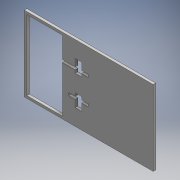
# Autodesk Inventor part: Lag2
Saved by Autodesk Inventor 2016 (Build 200138000, 138)
## iProperties
Created: 2016-12-11
Part Number: Lag2
Material: Generic
Document SubType Name: Modeling
Designer: Simon
Density: 1 g/cm^3
Appearance: Default
Author: Simon
Autodesk Inventor part; units mm, degrees
ref_plane "YZ Plane" through (0, 0, 0) normal (1, 0, 0) x (0, 1, 0)
ref_plane "XZ Plane" through (0, 0, 0) normal (0, 1, 0) x (-1, 0, 0)
ref_plane "XY Plane" through (0, 0, 0) normal (0, 0, 1) x (1, 0, 0)
sketch "Sketch1" plane through (0, 0, 0) normal (0, 1, 0) x (-1, 0, 0)
  line L0 (-50.5, 29.5) -> (50.5, 29.5)
  line L1 (50.5, 29.5) -> (50.5, -29.5)
  line L2 (50.5, -29.5) -> (-50.5, -29.5)
  line L3 (-50.5, -29.5) -> (-50.5, 29.5)
  line L4 (-50.5, 29.5) -> (50.5, -29.5) construction
  line L5 (50.5, 29.5) -> (-50.5, -29.5) construction
  line L6 (5.5, 16.6667) -> (10.5, 16.6667)
  line L7 (10.5, 6.6667) -> (5.5, 6.6667)
  line L8 (5.5, 6.6667) -> (5.5, 16.6667)
  line L9 (5.5, 16.6667) -> (10.5, 6.6667) construction
  line L10 (10.5, 16.6667) -> (5.5, 6.6667) construction
  line L11 (5.5, -16.6667) -> (10.5, -16.6667)
  line L12 (10.5, -6.6667) -> (5.5, -6.6667)
  line L13 (5.5, -16.6667) -> (10.5, -6.6667) construction
  line L14 (10.5, -16.6667) -> (5.5, -6.6667) construction
  line L15 (10.5, 10) -> (20.5, 10)
  line L16 (20.5, 11) -> (20.5, 9)
  line L17 (20.5, 9) -> (10.5, 9)
  line L18 (20.5, 11) -> (10.5, 11)
  line L19 (10.5, -10) -> (15.5, -10)
  line L20 (15.5, -9) -> (15.5, -11)
  line L21 (5.5, 10) -> (0.5, 10)
  line L22 (0.5, 11) -> (0.5, 9)
  line L23 (0.5, 11) -> (5.5, 11)
  line L24 (0.5, 9) -> (5.5, 9)
  line L25 (15.5, -11) -> (10.5, -11)
  line L26 (15.5, -9) -> (10.5, -9)
  line L27 (48.5, 27.5) -> (20.5, 27.5)
  line L28 (20.5, 27.5) -> (20.5, -27.5)
  line L29 (20.5, -27.5) -> (48.5, -27.5)
  line L30 (48.5, -27.5) -> (48.5, 27.5)
  line L31 (10.5, 16.6667) -> (10.5, 13.3333)
  line L32 (10.5, 13.3333) -> (10.5, 10)
  line L33 (10.5, 10) -> (10.5, 6.6667)
  line L34 (5.5, -16.6667) -> (5.5, -13.3333)
  line L35 (5.5, -13.3333) -> (5.5, -10)
  line L36 (5.5, -10) -> (5.5, -6.6667)
  line L37 (0.5, -11) -> (0.5, -9)
  line L38 (5.5, -10) -> (0.5, -10)
  line L39 (0.5, -11) -> (5.5, -11)
  line L40 (0.5, -9) -> (5.5, -9)
  line L41 (10.5, -16.6667) -> (10.5, -6.6667)
  line L42 (8, 11.6667) -> (8, -11.6667)
  line L43 (50.5, 0) -> (-50.5, 0)
  point P0 (0, 0)
  point P1 (0, 29.5)
  point P2 (0, -29.5)
  point P3 (8, 0)
  dimension "d0" = 101
  dimension "d1" = 59
  dimension "d4" = 5
  dimension "d5" = 10
  dimension "d6" = 10
  dimension "d7" = 2
  dimension "d8" = 5
  dimension "d14" = 20
  dimension "d15" = 2
  dimension "d16" = 2
  dimension "d17" = 55
  dimension "d18" = 2
  dimension "d19" = 28
  constraints: 88 end point, 21 equal length, 13 midpoint, 13 point on line, 11 horizontal, 8 vertical, 6 perpendicular, 3 collinear
  measures "d0" distance of L1.end L2.end
  measures "d1" distance of L0.end L1.end
  measures "d4" distance of L7.start L7.end
  measures "d5" distance of L6.end L7.start
  measures "d6" distance of L15.start L15.end
  measures "d7" distance of L16.start L16.end
  measures "d8" distance of L21.start L21.end
  measures "d14" distance between parallel lines of L19 L15
  measures "d15" distance between parallel lines of L2 L29
  measures "d16" distance between parallel lines of L0 L27
  measures "d17" distance of L29.end L27.start
  measures "d18" distance between parallel lines of L1 L30
  measures "d19" distance of L28.end L29.end
extrude "Extrusion4" add sketch "Sketch1" along normal blind 2 contours L0 L1 L43 L30 L27 L28 L18 L32 L31 L6 L8 L23 L22 L24 L7 L42 L3 | L43 L28 L29 L30 L1 L2 L3 | L42 L7 L33 L17 L28 L43
body "Solid4"
